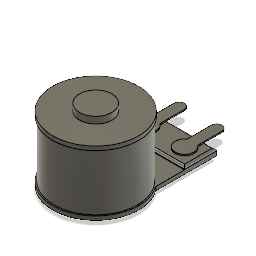
Smart Drop Target Left PBL-100-0043-00 (Autodesk Fusion 360 archive; units mm, degrees)
design "Coil SM1-26-600"
Autodesk Fusion 360 part; units mm, degrees
sketch "Sketch1" plane through (0, 0, 0) normal (0, 1, 0) x (1, 0, 0) in component "Coil Wiring"
  circle A0 centre (0, 0) radius 12.3031
  dimension "d1" = 24.6062
  measures "d1" diameter of A0
extrude "Extrude1" add sketch "Sketch1" along normal blind 16.6688 makes body 1 in component "Coil Wiring"
sketch "Sketch1 (2)" plane through (0, 0, 0) normal (0, 1, 0) x (1, 0, 0) in component "Plastic Top"
  circle A0 centre (50.8, -25.4) radius 12.7
  dimension "d4" = 25.4
  measures "d4" diameter of A0
extrude "Extrude1'" add sketch "Sketch1 (2)" along normal blind 1.1906 separate body makes body 2 in component "Plastic Top"
sketch "Sketch1 (3)" plane through (0, 0, 0) normal (0, 1, 0) x (1, 0, 0) in component "Plastic Bottom"
  circle A0 centre (25.4, -50.8) radius 12.7
  line L0 (25.4, -50.8) -> (25.4, -25.4)
  line L1 (25.4, -25.4) -> (15.0812, -25.4)
  line L2 (25.4, -25.4) -> (35.7187, -25.4)
  line L3 (35.7187, -25.4) -> (35.7187, -43.3964)
  line L4 (15.0812, -25.4) -> (15.0812, -43.3964)
  dimension "d7" = 25.4
  dimension "d8" = 25.4
  dimension "d9" = 10.3188
  measures "d7" diameter of A0
  measures "d9" distance of origin
extrude "Extrude1''" add sketch "Sketch1 (3)" along normal blind 1.1906 separate body makes body 3 in component "Plastic Bottom"
sketch "Sketch2" plane through (0, 1.1906, 0) normal (0, 1, 0) x (-1, 0, 0) in component "Plastic Bottom"
  line L0 (-35.7187, 25.4) -> (-15.0812, 25.4)
  line L1 (-15.0812, 25.4) -> (-15.0812, 43.3964)
  arc A0 (-15.0812, 43.3964) -> (-35.7187, 43.3964) centre (-25.4, 50.8) ccw
  line L2 (-35.7187, 43.3964) -> (-35.7187, 25.4)
  line L3 (-15.0812, 25.4) -> (-15.0812, 34.925)
  line L4 (-15.0812, 34.925) -> (-35.7187, 34.925)
extrude "Extrude2" add sketch "Sketch2" along normal blind 0.7937 contours L0 L1 L2 L3 L4 bodies 3 in component "Plastic Bottom"
fillet "Fillet1" radius 0.6604 4 edges at (35.7187, 1.9844, 30.1625) (25.4, 1.9844, 25.4) (25.4, 1.9844, 34.925) (15.0812, 1.9844, 30.1625) on bodies 3 in component "Plastic Bottom"
sketch "Sketch3" plane through (0, 1.9844, 0) normal (0, 1, 0) x (-1, 0, 0) in component "Plastic Bottom"
  line L0 (-15.7416, 26.0604) -> (-15.7416, 34.2646)
  line L1 (-15.7416, 34.2646) -> (-35.0583, 34.2646)
  line L2 (-35.0583, 34.2646) -> (-35.0583, 26.0604)
  line L3 (-35.0583, 26.0604) -> (-15.7416, 26.0604)
  line L4 (-15.0812, 25.4) -> (-15.0812, 34.925)
  line L5 (-35.7187, 34.925) -> (-35.7187, 25.4)
  circle A0 centre (-19.8437, 30.1625) radius 2.7781
  circle A1 centre (-30.9562, 30.1625) radius 2.7781
  line L6 (-18.2562, 20.6375) -> (-18.2562, 27.8826)
  line L7 (-21.4312, 20.6375) -> (-21.4312, 27.8826)
  line L8 (-29.3687, 20.6375) -> (-29.3687, 27.8826)
  line L9 (-32.5437, 20.6375) -> (-32.5437, 27.8826)
  arc A2 (-21.4312, 20.6375) -> (-18.2562, 20.6375) centre (-19.8437, 20.6375) ccw
  arc A3 (-32.5437, 20.6375) -> (-29.3687, 20.6375) centre (-30.9562, 20.6375) ccw
  dimension "d18" = 5.5563
  dimension "d19" = 5.5563
  measures "d18" diameter of A0
  measures "d19" diameter of A1
extrude "Extrude3" add sketch "Sketch3" along normal blind 0.3969 contours L3 L6 L7 A2 | L3 A0 L6 L7 | A0 | L3 L8 L9 A3 | L3 A1 L8 L9 | A1 bodies 3 in component "Plastic Bottom"
sketch "Sketch1 (4)" plane through (0, 0, 0) normal (0, 1, 0) x (1, 0, 0) in component "Core"
  circle A0 centre (25.4, -25.4) radius 4.7625
  dimension "d28" = 9.525
  measures "d28" diameter of A0
extrude "Extrude1'''" add sketch "Sketch1 (4)" along normal blind 22.225 separate body makes body 4 in component "Core"
sketch "Sketch4" plane through (0, 1.1906, 0) normal (0, 1, 0) x (-1, 0, 0) in component "Plastic Bottom"
  line L0 (-35.7187, 34.925) -> (-15.0812, 34.925)
  line L1 (-15.0812, 34.925) -> (-15.0812, 43.3964)
  arc A0 (-15.0812, 43.3964) -> (-35.7187, 43.3964) centre (-25.4, 50.8) ccw
  line L2 (-35.7187, 43.3964) -> (-35.7187, 34.925)
  circle A1 centre (-25.4, 50.8) radius 4.7625
  dimension "d31" = 9.525
  measures "d31" diameter of A1
extrude "Extrude4" cut sketch "Sketch4" against normal blind 1.1906 contours A1 bodies 3 in component "Plastic Bottom"
sketch "Sketch2 (2)" plane through (0, 1.1906, 0) normal (0, 1, 0) x (-1, 0, 0) in component "Plastic Top"
  circle A0 centre (-50.8, 25.4) radius 12.7
  circle A1 centre (-50.8, 25.4) radius 4.7625
  dimension "d34" = 9.525
  measures "d34" diameter of A1
extrude "Extrude2'" cut sketch "Sketch2 (2)" against normal blind 1.1906 contours A1 bodies 2 in component "Plastic Top"
sketch "Sketch2 (3)" plane through (0, 16.6688, 0) normal (0, 1, 0) x (-1, 0, 0) in component "Coil Wiring"
  circle A0 centre (0, 0) radius 12.3031
  circle A1 centre (0, 0) radius 4.7625
  dimension "d37" = 9.525
  measures "d37" diameter of A1
extrude "Extrude2''" cut sketch "Sketch2 (3)" against normal blind 16.6688 contours A1 bodies 1 in component "Coil Wiring"
component "Coil Wiring" placed x (1, 0, 0) y (0, 1, 0) z (0, 0, 1) at (0, 0, 0)
component "Plastic Top" placed x (1, 0, 0) y (0, 1, 0) z (0, 0, 1) at (-50.8, 16.6688, -25.4)
component "Plastic Bottom" placed x (1, 0, 0) y (0, 1, 0) z (0, 0, 1) at (-25.4, -1.1906, -50.8)
component "Core" placed x (1, 0, 0) y (0, 1, 0) z (0, 0, 1) at (-25.4, -2.3812, -25.4)
equation "d1 = ( 31 / 32 ) * 1 in"
equation "d2 = ( 21 / 32 ) * 1 in"
equation "d5 = ( 3 / 64 ) * 1 in"
equation "d9 = ( 13 / 32 ) * 1 in"
equation "d10 = ( 3 / 64 ) * 1 in"
equation "d13 = ( 1 / 32 ) * 1 in"
equation "d18 = ( 7 / 32 ) * 1 in"
equation "d19 = ( 7 / 32 ) * 1 in"
equation "d26 = ( 1 / 64 ) * 1 in"
equation "d28 = ( 3 / 8 ) * 1 in"
equation "d29 = ( 7 / 8 ) * 1 in"
equation "d31 = ( 3 / 8 ) * 1 in"
equation "d32 = ( -3 / 64 ) * 1 in"
equation "d34 = ( 3 / 8 ) * 1 in"
equation "d35 = ( -3 / 64 ) * 1 in"
equation "d37 = ( 3 / 8 ) * 1 in"
equation "d38 = ( -21 / 32 ) * 1 in"
